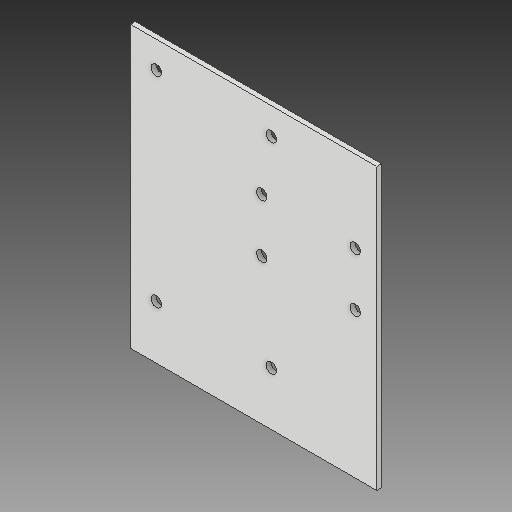
# Autodesk Inventor part: Part1
Saved by Autodesk Inventor 2018.3 (Build 223284000, 284)
## iProperties
Created: 2020-02-11
Part Number: Part1
Material: Generic
Document SubType Name: Modeling
Designer: Sam
Density: 1 g/cm^3
Appearance: Default
Mass: 24.3663 g
Surface Area: 315.871 cm^2
Volume: 24.3663 cm^3
Author: Sam
Autodesk Inventor part; units mm, degrees
ref_plane "YZ Plane" through (0, 0, 0) normal (1, 0, 0) x (0, 1, 0)
ref_plane "XZ Plane" through (0, 0, 0) normal (0, 1, 0) x (-1, 0, 0)
ref_plane "XY Plane" through (0, 0, 0) normal (0, 0, 1) x (1, 0, 0)
sketch "Sketch1" plane through (0, 0, 0) normal (0, 0, 1) x (1, 0, 0)
  line L0 (76.2, -65.8876) -> (-76.2, -65.8876)
  line L1 (-76.2, -65.8876) -> (-76.2, 65.8876)
  line L2 (-76.2, 65.8876) -> (40.8686, 65.8876)
  line L3 (76.2, 65.8876) -> (76.2, -65.8876)
  line L4 (76.2, -65.8876) -> (-76.2, 65.8876) construction
  line L5 (-76.2, -65.8876) -> (76.2, 65.8876) construction
  line L6 (-76.2, -65.8876) -> (-57.6516, -65.8876)
  line L7 (76.2, -65.8876) -> (57.6517, -65.8876)
  line L8 (40.8686, 65.8876) -> (40.8686, -65.8876)
  point P0 (0, 0)
  dimension "d10" = 131.7752
  dimension "d11" = 152.4
  dimension "d12" = 35.3314
  constraints: 18 end point, 3 point on line, 2 midpoint, 2 parallel, 2 perpendicular, 1 horizontal
  measures "d10" distance of L0.end L1.end
  measures "d11" distance of L1.end L3.start
  measures "d12" distance between parallel lines of L3 L8
extrude "Extrusion2" add sketch "Sketch1" along normal blind 2.286
sketch "Sketch2" plane through (0, 0, 0) normal (0, 0, -1) x (-1, 0, 0)
  circle A0 centre (13.7802, 28.6824) radius 2.0193 projected
  circle A1 centre (-30.6698, 28.6824) radius 2.0193 projected
  circle A2 centre (-30.6698, 3.2824) radius 2.0193 projected
  circle A3 centre (13.7802, 3.2824) radius 2.0193 projected
  point P0 (0, 0)
hole "Hole1" at (-13.7802, 3.2824, 0) at (30.6698, 3.2824, 0) at (30.6698, 28.6824, 0) at (-13.7802, 28.6824, 0) direction (0, 0, 1) diameter 4.9784 end through all clearance for "Flat Head Machine Screw (82)" size "#10" standard "Ansi Unified Screw Threads"
sketch "Sketch3" plane through (0, 0, 0) normal (0, 0, -1) x (-1, 0, 0)
  line L0 (-126.5936, 67.4624) -> (-126.5936, 42.0624) projected
  line L1 (-126.5936, 67.4624) -> (610.0064, 67.4624) projected
  line L2 (-126.5936, 42.0624) -> (610.0064, 42.0624) projected
  line L3 (-66.2686, -65.8876) -> (549.6814, -65.8876) projected
  line L4 (549.6814, -15.0876) -> (-66.2686, -15.0876) projected
  point P0 (0, 0)
  point P1 (63.9064, -40.4876)
  point P2 (9.2456, -40.4876)
  point P3 (63.9064, 54.7624)
  point P4 (9.2456, 54.7624)
  dimension "d21" = 190.5
  dimension "d22" = 0
  dimension "d23" = 25.4
  dimension "d24" = 12.7
  dimension "d25" = 25.4
  dimension "d26" = 12.7
  dimension "d27" = 135.8392
  dimension "d28" = 135.8392
  measures "d21" distance from line of L0 point (63.906, -40.488)
  measures "d22" horizontal distance of point (63.906, 54.762) point (63.906, -40.488)
  measures "d23" distance from line of L3 point (63.906, -40.488)
  measures "d24" distance from line of L1 point (63.906, 54.762)
  measures "d25" distance from line of L3 point (9.246, -40.488)
  measures "d26" distance from line of L1 point (9.246, 54.762)
  measures "d27" distance from line of L0 point (9.246, 54.762)
  measures "d28" distance from line of L0 point (9.246, -40.488)
hole "Hole2" at (-63.9064, -40.4876, 0) at (-9.2456, -40.4876, 0) at (-63.9064, 54.7624, 0) at (-9.2456, 54.7624, 0) direction (0, 0, 1) diameter 4.9784 end through all clearance for "Flat Head Machine Screw (82)" size "#10" standard "Ansi Unified Screw Threads"
sketch "Sketch4" plane through (0, 0, 0) normal (0, 0, -1) x (-1, 0, 0)
  line L0 (-40.8686, 65.8876) -> (76.2, 65.8876) projected
  line L1 (-40.8686, 65.8876) -> (76.2, 65.8876)
  line L2 (76.2, 65.8876) -> (76.2, 67.4624)
  line L3 (76.2, 67.4624) -> (-40.8686, 67.4624)
  line L4 (-40.8686, 67.4624) -> (-40.8686, 65.8876)
  line L5 (76.2, -65.8876) -> (76.2, 65.8876) projected
  point P0 (0, 0)
  dimension "d36" = 1.5748
  constraints: 8 end point, 2 parallel, 1 collinear, 1 horizontal, 1 perpendicular
  measures "d36" distance between parallel lines of L0 L3
extrude "Extrusion3" add sketch "Sketch4" against normal up to surface (2.286 mm away)
equation "\"d28\" = d27"
body "Solid2"
